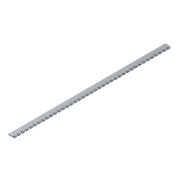
# Autodesk Inventor part: FE-00010-02
Saved by Autodesk Inventor 2012 (Build 160160000, 160)
## iProperties
Created: 2008-05-25
Part Number: FE-00010-02
Document SubType Name: Modeling
Designer: firstuser
Density: 1 g/cm^3
Mass: 150.764 g
Surface Area: 1057.55 cm^2
Volume: 150.764 cm^3
Material: Default
Author: firstuser
Autodesk Inventor part; units mm, degrees
ref_plane "YZ Plane" through (0, 0, 0) normal (1, 0, 0) x (0, 1, 0)
ref_plane "XZ Plane" through (0, 0, 0) normal (0, 1, 0) x (-1, 0, 0)
ref_plane "XY Plane" through (0, 0, 0) normal (0, 0, 1) x (1, 0, 0)
sketch "Sketch1" plane through (0, 0, 0) normal (0, 0, 1) x (1, 0, 0)
  line L0 (-41.275, 0) -> (-41.275, 3.175)
  line L1 (-41.275, 3.175) -> (-8.6743, 3.175)
  arc A0 (-3.175, 0) -> (-8.6743, 3.175) centre (-3.175, 6.35) ccw
  line L2 (-41.275, 0) -> (-3.175, 0)
  circle A1 centre (-3.175, 6.35) radius 3.175
  dimension "d0" = 6.35
  dimension "d1" = 38.1
  dimension "d2" = 3.175
  dimension "d3" = 6.35
  constraints: 6 end point, 2 centre point, 2 point on circle, 1 coincident, 1 perpendicular, 1 tangent, 1 vertical
  measures "d0" diameter of A1
  measures "d1" distance from line of A0.centre L0
  measures "d2" distance of L0.start L0.end
  measures "d3" radius of A0
extrude "Extrusion1" add sketch "Sketch1" along normal blind 990.6
sketch "Sketch2" plane through (-41.275, 0, 0) normal (0, -1, 0) x (1, 0, 0)
  line L0 (38.1, 990.6) -> (0, 990.6) projected
  line L1 (0, 0) -> (0, 990.6) projected
  line L2 (63.5, 977.9) -> (31.75, 977.9)
  line L3 (31.75, 977.9) -> (31.75, 965.2)
  line L4 (31.75, 965.2) -> (63.5, 965.2)
  line L5 (63.5, 965.2) -> (63.5, 977.9)
  dimension "d6" = 12.7
  dimension "d7" = 12.7
  dimension "d8" = 31.75
  dimension "d9" = 31.75
  constraints: 8 end point, 2 parallel, 1 horizontal, 1 perpendicular
  measures "d6" distance of L4.end L2.start
  measures "d7" distance between parallel lines of L0 L2
  measures "d8" distance between parallel lines of L3 L1
  measures "d9" distance of L2.start L2.end
extrude "Extrusion2" cut sketch "Sketch2" against normal blind 990.6
pattern_linear "Rectangular Pattern1" count 39 spacing 25.4 along (0, 0, -1) of "Extrusion2"
body "Solid1"
